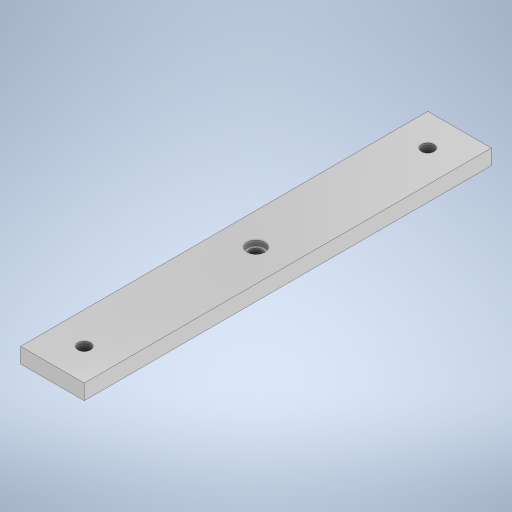
# Autodesk Inventor part: Suporte mesa
Saved by Autodesk Inventor 2023 (Build 270158000, 158)
## iProperties
Created: 2023-04-06
Part Number: Suporte mesa
Material: Aluminum 6061
Document SubType Name: Sheet Metal
Designer: 062190003
Density: 2.7 g/cm^3
Sheet Metal Rule: Default_mm
Appearance: Aluminum - Polished
Mass: 63.744 g
Surface Area: 103.975 cm^2
Volume: 23.6089 cm^3
Author: 062190003
Autodesk Inventor part; units mm, degrees
ref_plane "YZ Plane" through (0, 0, 0) normal (1, 0, 0) x (0, 1, 0)
ref_plane "XZ Plane" through (0, 0, 0) normal (0, 1, 0) x (-1, 0, 0)
ref_plane "XY Plane" through (0, 0, 0) normal (0, 0, 1) x (1, 0, 0)
sketch "Sketch1" plane through (0, 0, 0) normal (0, 1, 0) x (-1, 0, 0)
  line L0 (0, 0) -> (25, 0)
  line L1 (25, 0) -> (25, -160)
  line L2 (25, -160) -> (0, -160)
  line L3 (0, -160) -> (0, 0)
  dimension "d0" = 25
  dimension "d1" = 160
  constraints: 8 end point, 2 parallel, 1 horizontal, 1 perpendicular
  measures "d0" distance of L1.end L2.end
  measures "d1" distance of L0.end L1.end
extrude "Extrusion1" add sketch "Sketch1" along normal blind 6
sketch "Sketch2" plane through (0, 6, 0) normal (0, 1, 0) x (1, 0, 0)
  line L0 (-25, 160) -> (-25, 0) projected
  line L1 (-25, 0) -> (0, 0) projected
  line L2 (0, 160) -> (-25, 160) projected
  point P0 (-12.5, 12.5)
  point P1 (-12.5, 147.5)
  dimension "d4" = 25
  dimension "d5" = 160
  dimension "d6" = 12.5
  dimension "d7" = 12.5
  dimension "d8" = 12.5
  dimension "d9" = 12.5
  measures "d4" distance of L0.end L1.end
  measures "d5" distance of L0.start L0.end
  measures "d6" distance from line of L0 point (-12.5, 12.5)
  measures "d7" distance from line of L0 point (-12.5, 147.5)
  measures "d8" distance from line of L1 point (-12.5, 12.5)
  measures "d9" distance from line of L2 point (-12.5, 147.5)
hole "Hole1" at (-12.5, 6, -12.5) at (-12.5, 6, -147.5) direction (0, -1, 0) diameter 5 end through all
sketch "Esboço3" plane through (0, 6, 0) normal (0, 1, 0) x (1, 0, 0)
  line L0 (0, 160) -> (-25, 160) projected
  line L1 (0, 0) -> (0, 160) projected
  line L2 (-25, 160) -> (-25, 0) projected
  line L3 (-25, 0) -> (0, 0) projected
  point P0 (-12.5, 80)
  point P1 (-12.5, 0)
  dimension "d17" = 160
  dimension "d18" = 25
  dimension "d19" = 12.5
  dimension "d20" = 80
  constraints: 1 midpoint
  measures "d17" distance of L1.start L0.start
  measures "d18" distance of L0.start L0.end
  measures "d19" distance from line of L2 point (-12.5, 80)
  measures "d20" distance of point (-12.5, 0) point (-12.5, 80)
hole "Furo2" at (-12.5, 6, -80) direction (0, -1, 0) diameter 5 depth 6 tip angle 118 counterbore diameter 7 counterbore depth 2
thread "Rosca1" size "M5x0.8" class "6H" standard "ISO Metric profile" length 43.6
thread "Rosca2" size "M5x0.8" class "6H" standard "ISO Metric profile" length 15
equation "\"d6\" = 0.5 * d4"
equation "\"d7\" = d6"
equation "\"d9\" = d8"
equation "\"d15\" = Thickness"
equation "\"d19\" = 0.5 * d18"
equation "\"d20\" = 0.5 * d17"
equation "\"d26\" = Thickness"
equation "\"BendRadius\" = Thickness"
equation "\"BendReliefWidth\" = Thickness"
equation "\"BendReliefDepth\" = 0.5 * Thickness"
equation "\"CornerReliefSize\" = 4 * Thickness"
equation "\"MinimumRemnant\" = 2 * Thickness"
equation "\"TransitionRadius\" = BendRadius"
equation "\"JacobiRadiusSize\" = BendRadius"
equation "\"GapSize\" = Thickness"
equation "\"Thickness\" = 0.5"
body "Solid1"
